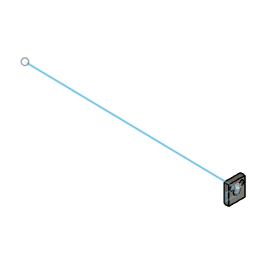
deneme (Autodesk Fusion 360 design; units mm, degrees)
Autodesk Fusion 360 part; units mm, degrees
sketch "Eskiz1" plane through (0, 0, 0) normal (1, 0, 0) x (0, 1, 0)
  line L0 (0, 80) -> (-70, 80)
  line L1 (-70, 80) -> (-70, 0)
  line L2 (-70, 0) -> (-70, -80)
  line L3 (-70, -80) -> (0, -80)
  line L4 (0, -80) -> (70, -80)
  line L5 (70, -80) -> (70, 80)
  line L6 (70, 80) -> (0, 80)
  circle A0 centre (-40, 40) radius 20
  circle A1 centre (40, 40) radius 20
  circle A2 centre (0, 0) radius 30
  line L7 (-50, -30) -> (46.201, -30)
  constraint horizontal L0
  constraint perpendicular L0 L1
  constraint perpendicular L0 L2
  constraint perpendicular L2 L3
  constraint perpendicular L2 L4
  constraint perpendicular L3 L5
  constraint perpendicular L5 L6
  constraint coincident A2.centre origin
sketch "Eskiz2" plane through (0, 0, 0) normal (1, 0, 0) x (0, 1, 0)
  line L0 (-50, -30) -> (-50, -70)
  line L1 (-50, -70) -> (50, -70)
  line L2 (50, -70) -> (50, -30)
  line L3 (50, -30) -> (44.9021, -30)
  line L4 (44.9021, -30) -> (50, -30)
  line L5 (50, -10) -> (-50, -10)
  line L6 (-50, -10) -> (-50, -30)
  constraint vertical L0
  constraint perpendicular L0 L1
  constraint perpendicular L1 L2
  constraint perpendicular L2 L3
  constraint perpendicular L2 L5
  constraint perpendicular L5 L6
extrude "Ekstrüde Et1" add sketch "Eskiz1" along normal blind 40
sketch "Eskiz3" plane through (0, 0, 0) normal (1, 0, 0) x (0, 1, 0)
  line L0 (50, -10) -> (50, -30)
  line L1 (50, -30) -> (50, -40)
  constraint vertical L0
  constraint parallel L0 L1
hole "Delik1" at (0, -1.2207, 36.0339) direction (1, 0, 0) diameter 20 depth 60 tip angle 118
sketch "Eskiz4" plane through (0, 0, 0) normal (0, 0, 1) x (1, 0, 0)
  line L0 (-1830, 50) -> (0, 16.9589)
